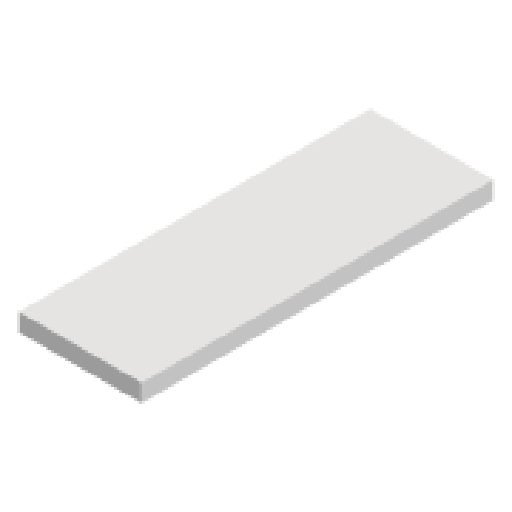
# Autodesk Inventor part: velcro piece
Saved by Autodesk Inventor 2025.2 (Build 292293000, 293)
## iProperties
Created: 2025-03-10
Part Number: velcro piece
Material: Generic
Document SubType Name: Modeling
Designer: Oscar
Density: 1 g/cm^3
Appearance: Default
Author: Oscar
Autodesk Inventor part; units mm, degrees
ref_plane "YZ Plane" through (0, 0, 0) normal (1, 0, 0) x (0, 1, 0)
ref_plane "XZ Plane" through (0, 0, 0) normal (0, 1, 0) x (-1, 0, 0)
ref_plane "XY Plane" through (0, 0, 0) normal (0, 0, 1) x (1, 0, 0)
sketch "Sketch1" plane through (0, 0, 0) normal (0, 1, 0) x (-1, 0, 0)
  line L0 (3.5, 10) -> (-3.5, 10)
  line L1 (-3.5, 10) -> (-3.5, -10)
  line L2 (-3.5, -10) -> (3.5, -10)
  line L3 (3.5, -10) -> (3.5, 10)
  point P0 (0, 0)
  point P1 (3.5, 0)
  point P2 (0, 10)
  dimension "d4" = 20
  dimension "d5" = 7
  constraints: 8 end point, 2 midpoint, 2 parallel, 1 horizontal, 1 horizontal alignment, 1 perpendicular, 1 vertical alignment
  measures "d4" distance of L2.end L0.start
  measures "d5" distance of L1.end L2.end
extrude "Extrusion1" add sketch "Sketch1" along normal blind 1
body "Solid1"
